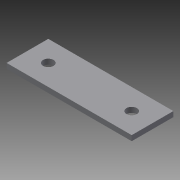
# Autodesk Inventor part: Spacer
Saved by Autodesk Inventor 2013 (Build 170138000, 138)
## iProperties
Created: 2013-07-16
Part Number: Spacer
Material: Aluminum 6061
Document SubType Name: Modeling
Designer: orange
Density: 1 g/cm^3
Author: orange
Autodesk Inventor part; units mm, degrees
ref_plane "YZ Plane" through (0, 0, 0) normal (1, 0, 0) x (0, 1, 0)
ref_plane "XZ Plane" through (0, 0, 0) normal (0, 1, 0) x (-1, 0, 0)
ref_plane "XY Plane" through (0, 0, 0) normal (0, 0, 1) x (1, 0, 0)
sketch "Sketch1" plane through (0, 0, 0) normal (0, 1, 0) x (-1, 0, 0)
  line L0 (-34.9521, -11.6688) -> (41.2479, -11.6688)
  line L1 (41.2479, -11.6688) -> (41.2479, 13.7312)
  line L2 (41.2479, 13.7312) -> (-34.9521, 13.7312)
  line L3 (-34.9521, 13.7312) -> (-34.9521, -11.6688)
  line L4 (-34.9521, -11.6688) -> (41.2479, 13.7312) construction
  line L5 (41.2479, -11.6688) -> (-34.9521, 13.7312) construction
  point P0 (0, 0)
  point P1 (3.1479, 1.0312)
  dimension "d0" = 76.2
  dimension "d2" = 25.4
  constraints: 12 end point, 2 midpoint, 2 parallel, 1 horizontal, 1 perpendicular
  measures "d0" distance of L0.start L0.end
  measures "d2" distance of L2.end L0.start
extrude "Extrusion1" add sketch "Sketch1" along normal blind 3.175
sketch "Sketch2" plane through (0, 3.175, 0) normal (0, 1, 0) x (1, 0, 0)
  line L0 (34.9521, 11.6688) -> (-41.2479, 11.6688) projected
  line L1 (-41.2479, 11.6688) -> (-41.2479, -13.7312) projected
  line L2 (34.9521, -13.7312) -> (34.9521, 11.6688) projected
  point P0 (0, 0)
  point P1 (-28.5479, -1.0312)
  point P2 (22.2521, -1.0312)
  dimension "d5" = 12.7
  dimension "d6" = 12.7
  dimension "d7" = 12.7
  dimension "d8" = 12.7
  measures "d5" distance from line of point (-28.548, -1.031) L0
  measures "d6" distance from line of point (22.252, -1.031) L0
  measures "d7" distance from line of L1 point (-28.548, -1.031)
  measures "d8" distance from line of point (22.252, -1.031) L2
hole "Hole1" at (-28.5479, 3.175, 1.0312) at (22.2521, 3.175, 1.0312) direction (0, -1, 0) diameter 6.35 end through all
body "Solid1"
